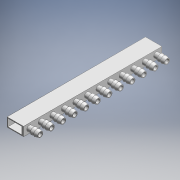
# Autodesk Inventor part: ManifoldExtension0
Saved by Autodesk Inventor 2018 (Build 220112000, 112)
## iProperties
Created: 2018-10-08
Part Number: ManifoldExtension0
Material: ABS Plastic
Document SubType Name: Modeling
Designer: Isaac Newcomb
Density: 1.06 g/cm^3
Appearance: Smooth - White
Width: 15.000 mm
FittingLength: 10.000 mm
myKeyWidth: 10.000 mm
myKeySpacing: 0.500 mm
Author: Isaac Newcomb
Autodesk Inventor part; units mm, degrees
ref_plane "YZ Plane" through (0, 0, 0) normal (1, 0, 0) x (0, 1, 0)
ref_plane "XZ Plane" through (0, 0, 0) normal (0, 1, 0) x (-1, 0, 0)
ref_plane "Silicone Fitting Plane" through (0, 0, -5.25) normal (0, 0, 1) x (1, 0, 0)
ref_plane "Cap Plane" through (0, 0, -126) normal (0, 0, 1) x (1, 0, 0)
sketch "Base Sketch" plane through (0, 0, 0) normal (0, 0, 1) x (1, 0, 0)
  line L0 (0, 0) -> (15, 0)
  line L1 (15, 0) -> (15, 8.1625)
  line L2 (15, 8.1625) -> (0, 8.1625)
  line L3 (0, 8.1625) -> (0, 0)
  line L4 (1.5, 1.5) -> (12, 1.5)
  line L5 (12, 1.5) -> (12, 6.6625)
  line L6 (12, 6.6625) -> (1.5, 6.6625)
  line L7 (1.5, 6.6625) -> (1.5, 1.5)
  dimension "Height" = 8.1625
  dimension "Width" = 15
  dimension "d1" = 1.5
  dimension "d2" = 1.5
  dimension "d3" = 1.5
  dimension "FittingWallWallThickness" = 3
  constraints: 16 end point, 4 parallel, 2 horizontal, 2 perpendicular
  measures "Height" distance of L2.end L0.start
  measures "Width" distance of L0.start L0.end
  measures "d1" distance between parallel lines of L3 L7
  measures "d2" distance between parallel lines of L2 L6
  measures "d3" distance between parallel lines of L4 L0
  measures "FittingWallWallThickness" distance between parallel lines of L1 L5
extrude "Base" add sketch "Base Sketch" against normal blind 126
sketch "Silicone Fitting Sketch" plane through (0, 0, -5.25) normal (0, 0, 1) x (1, 0, 0)
  line L0 (15, 4.0812) -> (25, 4.0812) construction
  line L1 (25, 4.0812) -> (25, 1.7)
  line L2 (25, 1.7) -> (22, 1)
  line L3 (22, 1) -> (22, 1.7)
  line L4 (22, 1.7) -> (19, 1)
  line L5 (19, 1) -> (19, 1.7)
  line L6 (19, 1.7) -> (15, 1.7)
  line L7 (15, 1.7) -> (15, 4.0812)
  line L8 (25, 1.7) -> (19, 1.7) construction
  line L9 (15, 2.2) -> (25, 2.2)
  line L10 (-5, 0) -> (30, 0) construction
  point P0 (0, 0)
  dimension "FittingLength" = 10
  dimension "FittingRadius" = 2.3813
  dimension "d4" = 0.5
  dimension "BarbHeight" = 0.7
  dimension "BarbLength" = 3
  dimension "d5" = 15
  dimension "FittingClearance" = 1
  constraints: 20 end point, 4 perpendicular, 3 parallel, 2 point on line, 1 collinear, 1 horizontal, 1 midpoint
  measures "FittingLength" distance of L0.start L0.end
  measures "FittingRadius" distance of L6.end L0.start
  measures "d4" distance between parallel lines of L6 L9
  measures "BarbHeight" distance of L2.end L3.end
  measures "BarbLength" horizontal distance of L3.end L4.end
  measures "d5" distance from line of point (0, 0) L7
  measures "FittingClearance" distance from line of L10 L4.end
revolve "Silicone Fitting" add sketch "Silicone Fitting Sketch" angle 360 about axis through (15, 4.0812, -5.25) along (1, 0, 0)
sketch "Airflow Cut Sketch" plane through (15, 4.0812, -5.25) normal (1, 0, 0) x (0, 0, -1)
  circle A0 centre (0, 0) radius 1.8812 projected
  point P0 (-5.25, -4.0812)
extrude "Airflow Cut" cut sketch "Airflow Cut Sketch" against normal up to surface (3 mm away)
pattern_linear "Fitting Repetitions" count 12 spacing 10.5 along (0, 0, -1) of "Silicone Fitting", "Airflow Cut"
sketch "Sketch22" plane through (0, 0, 0) normal (0, 0, 1) x (1, 0, 0)
  line L0 (0.75, 0.75) -> (13.5, 0.75)
  line L1 (13.5, 0.75) -> (13.5, 7.4125)
  line L2 (13.5, 7.4125) -> (0.75, 7.4125)
  line L3 (0.75, 7.4125) -> (0.75, 0.75)
  line L4 (1.5, 1.5) -> (12, 1.5)
  line L5 (12, 1.5) -> (12, 6.6625)
  line L6 (12, 6.6625) -> (1.5, 6.6625)
  line L7 (1.5, 6.6625) -> (1.5, 1.5)
  point P0 (0, 0)
  dimension "d141" = 0.75
  dimension "d142" = 0.75
  dimension "d143" = 6.6625
  dimension "d144" = 12.75
  dimension "d145" = 1.5
  dimension "d146" = 0.75
  dimension "d147" = 0.75
  dimension "d148" = 0.75
  constraints: 16 end point, 4 parallel, 2 horizontal, 2 perpendicular
  measures "d141" horizontal distance of L0.start point (0, 0)
  measures "d142" horizontal distance of point (0, 0) L0.start
  measures "d143" distance of L2.end L0.start
  measures "d144" distance of L0.start L0.end
  measures "d145" distance between parallel lines of L1 L5
  measures "d146" distance between parallel lines of L2 L6
  measures "d147" distance between parallel lines of L0 L4
  measures "d148" distance between parallel lines of L3 L7
extrude "Extrusion21" cut sketch "Sketch22" against normal blind 10.5
sketch "Sketch23" plane through (0, 0, -126) normal (0, 0, -1) x (-1, 0, 0)
  line L0 (-12, 1.5) -> (-12, 6.6625) projected
  line L1 (-12, 6.6625) -> (-1.5, 6.6625) projected
  line L2 (-1.5, 6.6625) -> (-1.5, 1.5) projected
  line L3 (-1.5, 1.5) -> (-12, 1.5) projected
  point P0 (0, 0)
extrude "Extrusion24" add sketch "Sketch23" against normal blind 1.5
equation "\"Height\" = 2 * FittingRadius + 2 * FittingClearance + 2 * BarbHeight"
equation "\"Width\" = ManifoldWidth"
equation "\"d1\" = WallThickness"
equation "\"d2\" = WallThickness"
equation "\"d3\" = WallThickness"
equation "\"FittingWallWallThickness\" = 2 * WallThickness"
equation "\"FittingLength\" = ManifoldFittingLength"
equation "\"d5\" = Width"
equation "\"d11\" = myKeyWidth + myKeySpacing"
equation "\"d141\" = 0.5 * WallThickness"
equation "\"d142\" = 0.5 * WallThickness"
equation "\"d143\" = Height - WallThickness"
equation "\"d144\" = -0.5 * WallThickness + Width - 0.5 * FittingWallWallThickness"
equation "\"d145\" = 0.5 * FittingWallWallThickness"
equation "\"d146\" = 0.5 * WallThickness"
equation "\"d147\" = 0.5 * WallThickness"
equation "\"d148\" = 0.5 * WallThickness"
equation "\"d149\" = KeyWidth + KeySpacing"
equation "\"d155\" = WallThickness"
equation "\"myKeyWidth\" = KeyWidth"
equation "\"myKeySpacing\" = KeySpacing"
equation "\"WallThickness\" = 1.5"
equation "\"d6\" = -0.5 * myKeyWidth - 0.5 * myKeySpacing"
equation "\"ManifoldWidth\" = 15"
equation "\"ManifoldFittingLength\" = 10"
equation "\"KeyWidth\" = 10"
equation "\"KeySpacing\" = 0.5"
body "Solid3"
